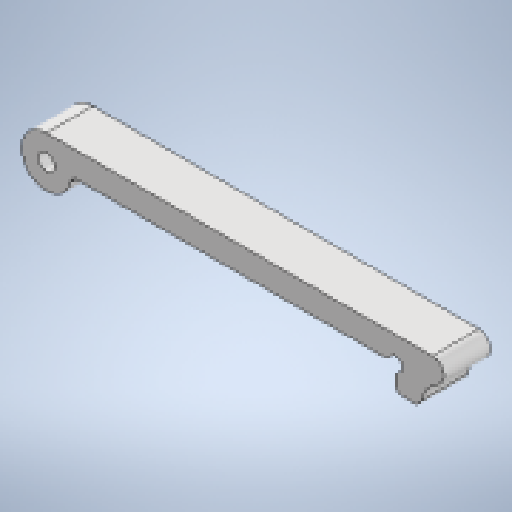
# Autodesk Inventor part: Lid
Saved by Autodesk Inventor 2023.2 (Build 272271000, 271)
## iProperties
Created: 2023-08-18
Part Number: Lid
Material: Generic
Document SubType Name: Modeling
Designer: Nathan Cai
Density: 1 g/cm^3
Appearance: Default
Author: Nathan Cai
Autodesk Inventor part; units mm, degrees
ref_plane "YZ Plane" through (0, 0, 0) normal (1, 0, 0) x (0, 1, 0)
ref_plane "XZ Plane" through (0, 0, 0) normal (0, 1, 0) x (-1, 0, 0)
ref_plane "XY Plane" through (0, 0, 0) normal (0, 0, 1) x (1, 0, 0)
sketch "Sketch1" plane through (0, 0, 0) normal (0, 0, 1) x (1, 0, 0)
  circle A0 centre (0, 0) radius 2.5
  circle A1 centre (0, 0) radius 7.5
  line L0 (-7.5, 0) -> (112.5, 0)
  line L1 (112.5, 0) -> (112.5, 7.5)
  line L2 (112.5, 7.5) -> (-7.5, 7.5)
  line L3 (-7.5, 7.5) -> (-7.5, 0)
  circle A2 centre (105, 0) radius 7.5 construction
  circle A3 centre (105, 0) radius 2
  line L4 (112.5, 7.5) -> (105, 7.5)
  line L5 (105, 7.5) -> (105, -7.5)
  line L6 (105, -7.5) -> (112.5, -7.5)
  line L7 (112.5, -7.5) -> (112.5, 7.5)
  circle A4 centre (116, 4) radius 3.5
  line L8 (112.5, 7.5) -> (116, 7.5)
  arc A5 (117.6076, 0.891) -> (112.5, -7.5) centre (121.9464, -7.5) ccw
  point P0 (7.5, 0)
  point P1 (103, 0)
  point P2 (105, -2)
  dimension "d1" = 15
  dimension "d3" = 15
  dimension "d0" = 5
  dimension "d2" = 120
  dimension "d4" = 4
  dimension "d5" = 7
  constraints: 18 end point, 4 centre point, 4 horizontal, 4 parallel, 4 point on circle, 4 tangent, 3 coincident, 2 perpendicular, 2 point on line, 2 vertical, 1 vertical alignment, 5 other
  measures "d0" diameter of A0
  measures "d2" distance of L2.end L1.end
  measures "d4" diameter of A3
  measures "d5" diameter of A4
extrude "Extrusion1" add sketch "Sketch1" along normal blind 15 contours L0 A1 A0 | A0 L0 A1 | A1 L2 L5 A3 L0 | L3 L2 A1 | L2 L1 L0 A3 L5 | A3 L0 L7 L6 L5 | L8 A4 L1 | A4 A5 L7 L1 | A4
fillet "Fillet1" radius 2 5 edges at (103, 0, 7.5) (105, -2, 7.5) (105, -7.5, 7.5) (112.5, -7.5, 7.5) (7.5, 0, 7.5)
fillet "Fillet2" radius 5 1 edges at (-7.5, 7.5, 7.5)
body "Solid1"
